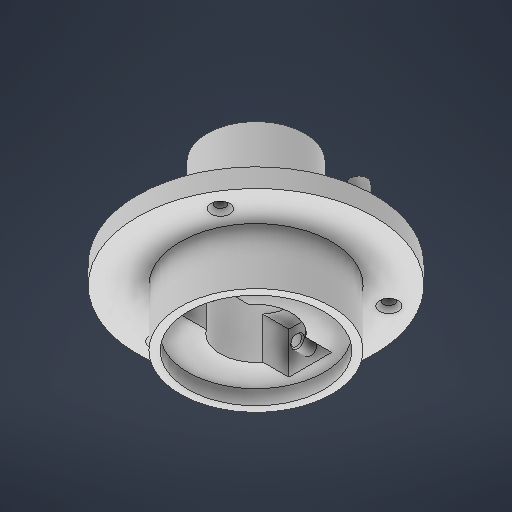
# Autodesk Inventor part: birdhouse_holder_v1
Saved by Autodesk Inventor 2026.2 (Build 302298000, 298)
## iProperties
Created: 2026-01-14
Part Number: birdhouse_holder_v1
Material: Generic
Document SubType Name: Modeling
Designer: User
Density: 1 g/cm^3
Appearance: Default
Author: User
Autodesk Inventor part; units mm, degrees
ref_plane "YZ Plane" through (0, 0, 0) normal (1, 0, 0) x (0, 1, 0)
ref_plane "XZ Plane" through (0, 0, 0) normal (0, 1, 0) x (-1, 0, 0)
sketch "Sketch1" plane through (0, 0, 0) normal (0, 1, 0) x (-1, 0, 0)
  circle A0 centre (0, 0) radius 13.25
  circle A1 centre (0, 0) radius 25.25
  circle A2 centre (0, 0) radius 28.25
  dimension "d0" = 26.5
  dimension "d1" = 12
  dimension "d2" = 3
  constraints: 3 centre point, 1 coincident
  measures "d0" diameter of A0
  measures "d1" radial gap between concentric circles of A0 A1
  measures "d2" radial gap between concentric circles of A1 A2
extrude "Extrusion1" add sketch "Sketch1" along normal blind 16 contours A2
extrude "Extrusion2" add sketch "Sketch1" along normal blind 10.5 contours A1
sketch "Sketch2" plane through (0, 10.5, 0) normal (0, 1, 0) x (1, 0, 0)
  line L0 (0, -8) -> (20.25, -8)
  line L1 (20.25, -8) -> (20.25, 8)
  line L2 (20.25, 8) -> (0, 8)
  line L3 (0, 8) -> (0, -8)
  circle A0 centre (0, 0) radius 13.25 projected
  line L4 (0, -8) -> (-20.25, -8)
  line L5 (-20.25, -8) -> (-20.25, 8)
  line L6 (-20.25, 8) -> (0, 8)
  point P0 (10.5623, 8)
  point P1 (10.5623, -8)
  point P2 (-10.5623, -8)
  point P3 (-10.5623, 8)
  dimension "d7" = 20.25
  dimension "d8" = 0
  dimension "d9" = 16
  constraints: 14 end point, 2 parallel, 2 symmetric about line, 1 horizontal, 1 midpoint, 1 perpendicular
  measures "d7" distance from line of L1 A0.centre
  measures "d8" distance of point (0, 0) point (0, 0)
  measures "d9" distance of L0.end L1.end
extrude "Extrusion3" cut sketch "Sketch2" against normal blind 10.5 contours A0 L2 L1 L0 | L4 L5 L6 A0
sketch "Sketch3" plane through (-20.25, 10.5, 8) normal (1, 0, 0) x (0, 0, -1)
  circle A0 centre (8, -5.25) radius 2.49
  line L0 (0, 0) -> (16, 0) projected
  line L1 (0, 0) -> (0, -10.5) projected
  point P0 (8, -10.5)
  point P1 (8, 0)
  point P2 (0, -5.25)
  dimension "d12" = 4.98
  dimension "d13" = 0
  dimension "d14" = 0
  constraints: 2 midpoint, 1 centre point
  measures "d12" diameter of A0
  measures "d13" horizontal distance of point (8, 0) A0.centre
  measures "d14" vertical distance of point (0, -5.25) A0.centre
extrude "Extrusion4" add sketch "Sketch3" along normal blind 5.25
chamfer "Chamfer1" distance 0.5 angle 45 1 edges at (-15, 5.25, 2.49)
ref_plane "Work Plane1" through (0, 0, 0) normal (1, 0, 0) x (0, 0, -1)
mirror "Mirror1" about plane through (0, 0, 0) normal (1, 0, 0) of "Extrusion4", "Chamfer1"
sketch "Sketch4" plane through (0, 0, 0) normal (0, -1, 0) x (1, 0, 0)
  circle A0 centre (0, 0) radius 28.25
  line L0 (20.25, -8) -> (10.5623, -8) projected
  line L1 (-20.25, 8) -> (-10.5623, 8) projected
  line L2 (20.25, -8) -> (-20.25, -8)
  line L3 (-20.25, -8) -> (-20.25, 8)
  line L4 (-20.25, 8) -> (20.25, 8)
  line L5 (20.25, 8) -> (20.25, -8)
  circle A1 centre (0, 0) radius 13.25
  point P0 (10.5623, 8)
  point P1 (-10.5623, -8)
  constraints: 8 end point, 2 centre point, 2 coincident, 2 parallel, 1 horizontal, 1 perpendicular
extrude "Extrusion5" add sketch "Sketch4" along normal blind 5
sketch "Sketch5" plane through (0, -5, 0) normal (0, -1, 0) x (1, 0, 0)
  circle A0 centre (0, 0) radius 13.25
  circle A1 centre (0, 0) radius 18.25
  circle A2 centre (0, 0) radius 44.25
  dimension "d22" = 5
  dimension "d23" = 26
  constraints: 3 centre point, 1 coincident
  measures "d22" radial gap between concentric circles of A0 A1
  measures "d23" radial gap between concentric circles of A1 A2
extrude "Extrusion6" add sketch "Sketch5" along normal blind 40 contours A1
extrude "Extrusion7" add sketch "Sketch5" along normal blind 7 contours A2
sketch "Sketch6" plane through (0, -12, 0) normal (0, -1, 0) x (1, 0, 0)
  circle A0 centre (0, 38.325) radius 3.15
  point P0 (0, 0)
  dimension "d28" = 6.3
  dimension "d29" = 38.325
  constraints: 1 centre point
  measures "d28" diameter of A0
  measures "d29" distance of point (0, 0) A0.centre
extrude "Extrusion8" add sketch "Sketch6" along normal blind 7
sketch "Sketch7" plane through (0, -12, 0) normal (0, -1, 0) x (1, 0, 0)
  circle A0 centre (0, 0) radius 28.25 projected
  line L0 (0, -28.25) -> (0, -44.25)
  circle A1 centre (0, 0) radius 44.25 projected
  circle A2 centre (0, -36.25) radius 2
  circle A3 centre (31.3934, 18.125) radius 2
  circle A4 centre (-31.3934, 18.125) radius 2
  dimension "d32" = 4
  dimension "d35" = 360
  constraints: 3 centre point, 2 end point, 2 vertical alignment, 1 midpoint, 1 vertical, 9 other
  measures "d32" diameter of A2
extrude "Extrusion9" cut sketch "Sketch7" against normal blind 7 contours A2 L0 | L0 A2 | A3 | A4
chamfer "Chamfer2" distance 1.5 angle 45 3 edges at (29.3934, -5, 18.125) (-33.3934, -5, 18.125) (-2, -5, -36.25)
body "Solid1"
